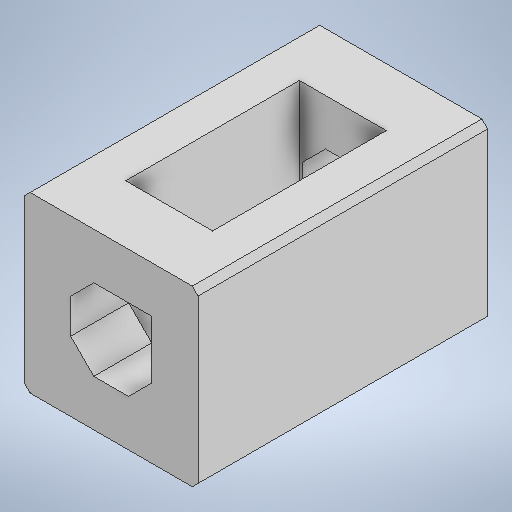
# Autodesk Inventor part: Test Square
Saved by Autodesk Inventor 2026.2 (Build 302298010, 298A)
## iProperties
Created: 2026-05-07
Part Number: Test Square
Material: Generic
Document SubType Name: Modeling
Designer: piete
Density: 1 g/cm^3
Appearance: Default
Author: piete
Autodesk Inventor part; units mm, degrees
ref_plane "YZ Plane" through (0, 0, 0) normal (1, 0, 0) x (0, 1, 0)
ref_plane "XZ Plane" through (0, 0, 0) normal (0, 1, 0) x (-1, 0, 0)
ref_plane "XY Plane" through (0, 0, 0) normal (0, 0, 1) x (1, 0, 0)
sketch "Sketch1" plane through (0, 0, 0) normal (0, 1, 0) x (-1, 0, 0)
  line L0 (7.5, 12.5) -> (-7.5, 12.5)
  line L1 (-7.5, 12.5) -> (-7.5, -12.5)
  line L2 (-7.5, -12.5) -> (7.5, -12.5)
  line L3 (7.5, -12.5) -> (7.5, 12.5)
  line L4 (3.75, 7.5) -> (-3.75, 7.5)
  line L5 (-3.75, 7.5) -> (-3.75, -7.5)
  line L6 (-3.75, -7.5) -> (3.75, -7.5)
  line L7 (3.75, -7.5) -> (3.75, 7.5)
  point P0 (0, 0)
  dimension "d0" = 15
  dimension "d1" = 25
  dimension "d2" = 12.5
  dimension "d3" = 7.5
  dimension "d4" = 7.5
  dimension "d5" = 15
  dimension "d6" = 3.75
  dimension "d7" = 7.5
  constraints: 16 end point, 4 parallel, 2 horizontal, 2 perpendicular
  measures "d0" distance of L2.end L1.end
  measures "d1" distance of L1.end L0.end
  measures "d2" distance from line of point (0, 0) L2
  measures "d3" distance from line of point (0, 0) L3
  measures "d4" distance of L6.end L5.end
  measures "d5" distance of L5.end L4.end
  measures "d6" distance from line of L5 point (0, 0)
  measures "d7" distance from line of point (0, 0) L6
extrude "Extrusion1" add sketch "Sketch1" along normal blind 15
sketch "Sketch2" plane through (-7.5, 0, 12.5) normal (0, 0, 1) x (1, 0, 0)
  line L0 (4, 11) -> (11, 11)
  line L1 (11, 11) -> (11, 4)
  line L2 (11, 4) -> (4, 4)
  line L3 (4, 4) -> (4, 11)
  line L4 (0, 0) -> (15, 0) projected
  line L5 (15, 0) -> (15, 15) projected
  point P0 (7.5, 0)
  point P1 (7.5, 0)
  point P2 (7.5, 4)
  point P3 (15, 7.5)
  point P4 (11, 7.5)
  dimension "d10" = 7
  dimension "d11" = 7
  dimension "d12" = 0
  dimension "d13" = 0
  constraints: 8 end point, 4 midpoint, 2 parallel, 1 horizontal, 1 perpendicular
  measures "d10" distance of L1.end L2.end
  measures "d11" distance of L0.end L1.end
  measures "d12" horizontal distance of point (7.5, 0) point (7.5, 4)
  measures "d13" vertical distance of point (15, 7.5) point (11, 7.5)
extrude "Extrusion2" cut sketch "Sketch2" against normal through all
chamfer "Chamfer1" distance 2 angle 45 7 edges at (-3.5, 11, 10) (-3.5, 4, 10) (3.5, 4, 10) (-3.5, 4, -10) (3.5, 4, -10) (3.5, 11, -10) (-3.5, 11, -10)
chamfer "Chamfer2" distance 0.5 angle 45 4 edges at (7.5, 0, 0) (7.5, 15, 0) (-7.5, 15, 0) (-7.5, 0, 0)
equation "\"d2\" = 0.5 * d1"
equation "\"d3\" = 0.5 * d0"
equation "\"d6\" = 0.5 * d4"
equation "\"d7\" = 0.5 * d5"
body "Solid1"
